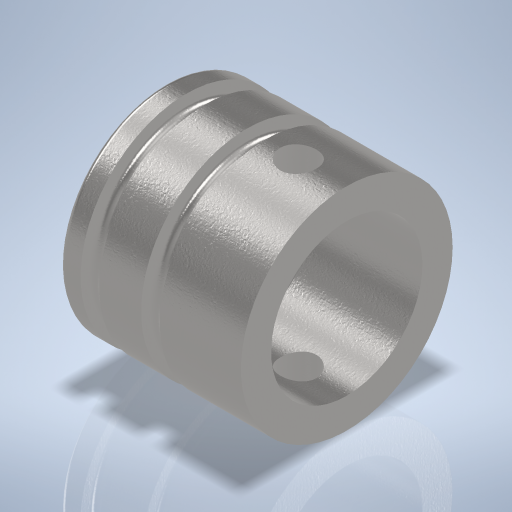
# Autodesk Inventor part: Kolben
Saved by Autodesk Inventor 2024 (Build 280153000, 153)
## iProperties
Created: 2024-03-01
Part Number: Kolben
Material: Stahl, galvanisiert
Document SubType Name: Modeling
Designer: ffogue
Density: 7.85 g/cm^3
Appearance: Galvanisiert
Author: ffogue
Autodesk Inventor part; units mm, degrees
ref_plane "YZ Plane" through (0, 0, 0) normal (1, 0, 0) x (0, 1, 0)
ref_plane "XZ Plane" through (0, 0, 0) normal (0, 1, 0) x (-1, 0, 0)
sketch "Skizze1" plane through (0, 0, 0) normal (0, 0, 1) x (1, 0, 0)
  line L0 (0, 0) -> (30, 0)
  line L1 (0, 0) -> (0, 17.5)
  line L2 (0, 17.5) -> (3.5, 17.5)
  line L3 (3.5, 17.5) -> (3.5, 15.005)
  line L4 (3.5, 15.005) -> (6.6, 15.005)
  line L5 (6.6, 15.005) -> (6.6, 17.5)
  line L6 (6.6, 17.5) -> (13.5, 17.5)
  line L7 (13.5, 17.5) -> (13.5, 15.005)
  line L8 (13.5, 15.005) -> (16.6, 15.005)
  line L9 (16.6, 15.005) -> (16.6, 17.5)
  line L10 (16.6, 17.5) -> (30, 17.5)
  line L11 (30, 17.5) -> (30, 0)
  point P0 (13.5, 16.2525)
  dimension "d0" = 35
  dimension "d1" = 30.01
  dimension "d3" = 16.5
  dimension "d4" = 26.5
  dimension "d5" = 30
  dimension "d6" = 3.1
  constraints: 24 end point, 6 perpendicular, 6 point on line, 1 coincident, 1 collinear, 1 horizontal, 1 midpoint, 1 vertical
  measures "d0" diameter of L10 L0
  measures "d1" diameter of L4 L0
  measures "d3" distance between parallel lines of L7 L11
  measures "d4" distance between parallel lines of L3 L11
  measures "d5" distance between parallel lines of L11 L1
  measures "d6" distance from line of L9 point (13.5, 16.253)
revolve "Umdrehung1" add sketch "Skizze1" angle 360 about axis through (0, 0, 0) along (1, 0, 0)
sketch "Skizze2" plane through (30, 0, 0) normal (1, 0, 0) x (0, 0, -1)
  circle A0 centre (0, 0) radius 17.5 projected
  constraints: 1 coincident
hole "Bohrung1" at (30, 0, 0) direction (-1, 0, 0) diameter 25 depth 17.5 tip angle 118
fillet "Rundung1" radius 1 1 edges at (0, -17.5, 0)
fillet "Rundung2" radius 1 2 edges at (3.5, -15.005, 0) (13.5, -15.005, 0)
ref_plane "Arbeitsebene13" through (0, 0, 0) normal (0, 0, 1) x (1, 0, 0)
sketch "Skizze17" plane through (0, 0, 0) normal (0, 0, 1) x (1, 0, 0)
  line L0 (30, 12.5) -> (30, -12.5) projected
  point P0 (0, 0)
  point P1 (22, 0)
  dimension "d51" = 8
  constraints: 1 horizontal alignment
  measures "d51" distance from line of L0 point (22, 0)
hole "Bohrung4" at (22, 0, 0) direction (0, 0, -1) diameter 5.98 end through all both
